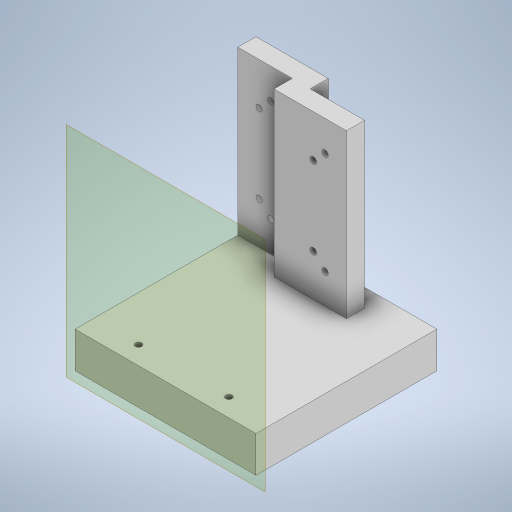
# Autodesk Inventor part: container_mid_1
Saved by Autodesk Inventor 2023 (Build 270158000, 158)
## iProperties
Created: 2022-11-30
Part Number: container_mid_1
Material: Genérico
Document SubType Name: Modeling
Designer: inigo
Density: 1 g/cm^3
Appearance: Valor por defecto
Author: inigo
Autodesk Inventor part; units mm, degrees
ref_plane "YZ Plane" through (0, 0, 0) normal (1, 0, 0) x (0, 1, 0)
ref_plane "XZ Plane" through (0, 0, 0) normal (0, 1, 0) x (-1, 0, 0)
ref_plane "XY Plane" through (0, 0, 0) normal (0, 0, 1) x (1, 0, 0)
sketch "Boceto1" plane through (0, 0, 0) normal (0, 0, 1) x (1, 0, 0)
  line L0 (-15, 45) -> (15, 45)
  line L1 (15, 45) -> (15, -45)
  line L2 (15, -45) -> (-15, -45)
  line L3 (-15, -45) -> (-15, 45)
  line L4 (-15, 45) -> (15, -45) construction
  line L5 (15, 45) -> (-15, -45) construction
  point P0 (0, 0)
  dimension "d0" = 30
  dimension "d1" = 90
  constraints: 12 end point, 2 midpoint, 2 parallel, 1 horizontal, 1 perpendicular
  measures "d0" distance of L1.end L2.end
  measures "d1" distance of L0.end L1.end
extrude "Extrusión1" add sketch "Boceto1" along normal blind 10
sketch "Boceto2" plane through (0, 0, 10) normal (0, 0, 1) x (1, 0, 0)
  line L0 (15, 45) -> (15, -45)
  line L1 (5, 30) -> (5, 20)
  line L2 (-5, 30) -> (5, 30)
  line L3 (5, 20) -> (-5, 30) construction
  line L4 (5, 20) -> (-5, 20)
  line L5 (-5, 20) -> (5, 30) construction
  line L6 (-5, 20) -> (-5, 30)
  line L7 (24, 0) -> (9, 0)
  line L8 (-15, -45) -> (15, -45)
  line L9 (5, 25) -> (5.4102, 25)
  circle A0 centre (-3.25, 21.75) radius 1.75
  circle A1 centre (3.25, 28.25) radius 1.75
  line L10 (5, -20) -> (-5, -20)
  circle A2 centre (-3.25, -21.75) radius 1.75
  line L11 (5, -25) -> (5.4102, -25)
  line L12 (5, -30) -> (5, -20)
  line L13 (-5, -30) -> (5, -30)
  line L14 (5, -20) -> (-5, -30) construction
  line L15 (-5, -20) -> (5, -30) construction
  line L16 (-5, -20) -> (-5, -30)
  circle A3 centre (3.25, -28.25) radius 1.75
  line L17 (-15, -45) -> (-15, 45)
  line L18 (15, -45) -> (15, 45) projected
  line L19 (-15, -45) -> (15, -45) projected
  line L20 (-15, 45) -> (15, 45)
  line L21 (-3.25, 28.25) -> (3.25, 21.75)
  line L22 (-3.25, 21.75) -> (3.25, 28.25)
  point P0 (0, 0)
  point P1 (-113, 215)
  point P2 (-5, 25)
  point P3 (-3.25, -21.75)
  point P4 (3.25, -28.25)
  point P5 (-143, 115)
  point P6 (-3.25, -21.75)
  point P7 (-5, -25)
  point P8 (3.25, -28.25)
  point P9 (0, 25)
  point P10 (0, -25)
  dimension "d4" = 1.75
  dimension "d5" = 1.75
  dimension "d6" = 1.75
  dimension "d7" = 1.75
  dimension "d8" = 10
  dimension "d9" = 10
  dimension "d10" = 10
  dimension "d11" = 15
  dimension "d12" = 0
  dimension "d13" = 30
  dimension "d14" = 0
  dimension "d15" = 90
  dimension "d16" = 15
  constraints: 38 end point, 11 symmetric about line, 4 centre point, 4 horizontal, 4 midpoint, 2 parallel, 1 perpendicular, 6 other
  measures "d4" distance from line of L2 L22.end
  measures "d5" distance from line of L1 L22.end
  measures "d6" distance from line of L6 L22.start
  measures "d7" distance from line of L4 L22.start
  measures "d8" distance between parallel lines of L4 L2
  measures "d9" distance between parallel lines of L1 L6
  measures "d10" distance between parallel lines of L17 L6
  measures "d12" horizontal extent of L18
  measures "d14" vertical extent of L19
  measures "d16" distance between parallel lines of L20 L2
hole "Agujero1" at (3.25, 28.25, 10) at (-3.25, 21.75, 10) at (-3.25, -21.75, 10) at (3.25, -28.25, 10) direction (0, 0, -1) diameter 3.5 end through all
sketch "Boceto3" plane through (-15, -45, 0) normal (-1, 0, 0) x (0, 0, 1)
  line L0 (0, 0) -> (0, 90) projected
  line L1 (0, 90) -> (20, 90)
  line L2 (20, 90) -> (20, 0)
  line L3 (20, 0) -> (0, 0)
  line L4 (0, 0) -> (0, 90)
  point P0 (0, 45)
  dimension "d24" = 20
  dimension "d25" = 90
  constraints: 8 end point, 2 parallel, 1 horizontal, 1 perpendicular
  measures "d24" distance of L2.end L3.end
  measures "d25" distance of L1.end L2.end
extrude "Extrusión2" add sketch "Boceto3" along normal blind 10
sketch "Boceto4" plane through (-25, -45, 0) normal (-1, 0, 0) x (0, 0, 1)
  line L0 (20, 90) -> (10, 90) projected
  line L1 (10, 0) -> (10, 90) projected
  line L2 (20, 90) -> (10, 90)
  line L3 (10, 90) -> (10, 0)
  line L4 (10, 0) -> (20, 0)
  line L5 (20, 0) -> (20, 90)
  point P0 (0, 45)
  constraints: 8 end point, 2 parallel, 1 horizontal, 1 perpendicular
extrude "Extrusión3" add sketch "Boceto4" along normal blind 30
sketch "Boceto5" plane through (-15, -45, 20) normal (0, 0, 1) x (1, 0, 0)
  line L0 (-40, 0) -> (-70, 90)
  line L1 (-70, 90) -> (-40, 0)
  line L2 (-20, 75) -> (-20, 65)
  line L3 (-30, 75) -> (-20, 75)
  line L4 (-20, 65) -> (-30, 75) construction
  line L5 (-20, 65) -> (-30, 65)
  line L6 (-30, 65) -> (-20, 75) construction
  circle A0 centre (-28.25, 66.75) radius 1.75
  line L7 (-30, 65) -> (-30, 75)
  circle A1 centre (-21.75, 73.25) radius 1.75
  line L8 (-40, -20) -> (-40, 90)
  line L9 (-55, 45) -> (-143, 45)
  line L10 (-20, 25) -> (-30, 25)
  circle A2 centre (-28.25, 23.25) radius 1.75
  line L11 (-20, 15) -> (-20, 25)
  line L12 (-20, 25) -> (-30, 15) construction
  line L13 (-30, 25) -> (-20, 15) construction
  line L14 (-30, 25) -> (-30, 15)
  line L15 (-30, 15) -> (-20, 15)
  circle A3 centre (-21.75, 16.75) radius 1.75
  line L16 (-70, 0) -> (-40, 0)
  line L17 (0, 0) -> (-40, 0) projected
  line L18 (-40, 90) -> (-70, 90)
  line L19 (-40, 0) -> (-40, 90) projected
  point P0 (15, 45)
  point P1 (-30, 70)
  point P2 (-20, 70)
  point P3 (-20, 20)
  point P4 (-30, 20)
  point P5 (-55, 0)
  point P6 (-55, 90)
  dimension "d30" = 3.5
  dimension "d31" = 1.75
  dimension "d32" = 1.75
  dimension "d33" = 1.75
  dimension "d34" = 1.75
  dimension "d35" = 10
  dimension "d36" = 10
  dimension "d38" = 10
  dimension "d39" = -41.1096
  dimension "d40" = 15
  dimension "d41" = 0
  dimension "d42" = 15
  dimension "d43" = 90
  dimension "d45" = 0
  constraints: 34 end point, 8 symmetric about line, 5 midpoint, 4 centre point, 3 equal length, 3 horizontal, 1 perpendicular, 5 other
  measures "d30" diameter of A1
  measures "d31" distance from line of L3 A1.centre
  measures "d32" distance from line of L2 A1.centre
  measures "d33" distance from line of L7 A0.centre
  measures "d34" distance from line of L5 A0.centre
  measures "d35" distance between parallel lines of L5 L3
  measures "d36" distance between parallel lines of L2 L7
  measures "d38" length of L7
  measures "d39" distance from line of L0 point (-20, 70)
  measures "d40" distance between parallel lines of L16 L15
  measures "d41" distance from line of L17 point (-55, 0)
  measures "d42" distance between parallel lines of L18 L3
  measures "d43" distance from line of L16 point (-55, 90)
  measures "d45" horizontal extent of L19
hole "Agujero2" at (-36.75, 28.25, 20) at (-43.25, 21.75, 20) at (-43.25, -21.75, 20) at (-36.75, -28.25, 20) direction (0, 0, -1) diameter 3.5 end through all
sketch "Boceto6" plane through (-15, -45, 20) normal (0, 0, 1) x (1, 0, 0)
  line L0 (-10, 0) -> (-40, 0) projected
  line L1 (-40, 0) -> (60, 0)
  line L2 (60, 0) -> (60, -20)
  line L3 (60, -20) -> (-40, -20)
  line L4 (-40, -20) -> (-40, 0)
  point P0 (15, 45)
  dimension "d53" = 20
  constraints: 8 end point, 2 parallel, 1 horizontal, 1 perpendicular
  measures "d53" distance of L1.end L2.end
extrude "Extrusión4" add sketch "Boceto6" against normal blind 100
mirror "Simetría1" about plane through (-5, -55, -80) normal (0, 0, -1) of "Extrusión1", "Agujero1", "Extrusión2", "Agujero2", "Extrusión3", "Extrusión4"
ref_plane "Plano de trabajo2" through (45, -65, -80) normal (0, 0, -1) x (-1, 0, 0)
sketch "Boceto7" plane through (-15, -45, 20) normal (0, 1, 0) x (1, 0, 0)
  line L0 (30, 115) -> (30, 85)
  circle A0 centre (35, 90) radius 1.75
  line L1 (30, 85) -> (40, 85)
  line L2 (35, 110) -> (35, 90)
  circle A1 centre (35, 110) radius 1.75
  line L3 (40, 115) -> (30, 85) construction
  line L4 (40, 115) -> (30, 115)
  line L5 (30, 115) -> (40, 85) construction
  line L6 (40, 85) -> (40, 115)
  line L7 (60, 0) -> (60, 200) projected
  line L8 (-40, 0) -> (60, 0) projected
  line L9 (10, 0) -> (10, 134.4524)
  line L10 (-10, 115) -> (-10, 85)
  circle A2 centre (-15, 110) radius 1.75
  line L11 (-20, 115) -> (-10, 115)
  circle A3 centre (-15, 90) radius 1.75
  line L12 (-10, 85) -> (-20, 85)
  line L13 (-20, 115) -> (-10, 85) construction
  line L14 (-10, 115) -> (-20, 85) construction
  line L15 (-20, 85) -> (-20, 115)
  line L16 (-15, 110) -> (-15, 90)
  point P0 (15, 20)
  point P1 (189.1833, 40)
  point P2 (35, 115)
  point P3 (-85.8367, 100)
  point P4 (235.02, 100)
  point P5 (-15, 115)
  dimension "d56" = 5
  dimension "d57" = 5
  dimension "d58" = 3.5
  dimension "d59" = 5
  dimension "d60" = 5
  dimension "d61" = 10
  dimension "d62" = 30
  dimension "d64" = 20
  constraints: 28 end point, 7 symmetric about line, 4 centre point, 2 midpoint, 1 vertical, 5 other
  measures "d56" distance from line of L0 L2.start
  measures "d57" distance of point (35, 115) L2.start
  measures "d58" diameter of A0
  measures "d60" distance from line of L0 L2.end
  measures "d61" distance between parallel lines of L0 L6
  measures "d64" distance between parallel lines of L6 L7
hole "Agujero3" at (-30, -45, -90) at (-30, -45, -70) at (20, -45, -90) at (20, -45, -70) direction (0, -1, 0) diameter 3.5 end through all
split "Dividir1" plane through (45, -65, -80) removes the side toward (0, 0, 1)
